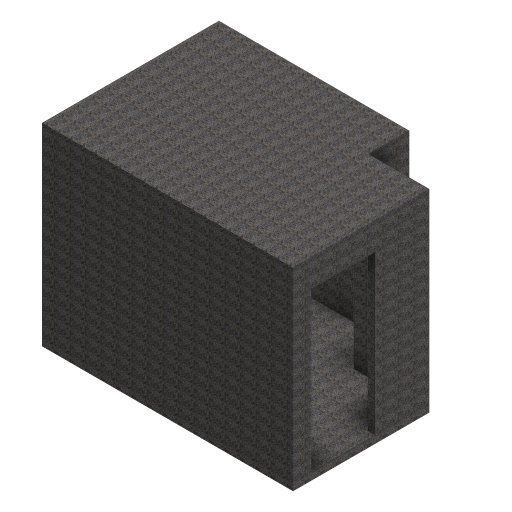
# Autodesk Inventor part: room
Saved by Autodesk Inventor 2023 (Build 270158000, 158)
## iProperties
Created: 2022-09-09
Part Number: room
Material: 混凝土
Document SubType Name: Modeling
Designer: byfbi
Density: 2.40731 g/cm^3
Appearance: 外露骨料 - 粗糙
Author: byfbi
Autodesk Inventor part; units mm, degrees
sketch "草图1" plane through (0, 0, 0) normal (0, 1, 0) x (-1, 0, 0)
  line L0 (0, 0) -> (0, 2400)
  line L1 (0, 2400) -> (-3500, 2400)
  line L2 (-3500, 2400) -> (-3500, 600)
  line L3 (-3500, 600) -> (-2600, 600)
  line L4 (-2600, 600) -> (-2600, 0)
  line L5 (-2600, 0) -> (0, 0)
  line L6 (110, 2510) -> (110, -110)
  line L7 (110, -110) -> (-2710, -110)
  line L8 (-2710, -110) -> (-2710, 490)
  line L9 (-2710, 490) -> (-3610, 490)
  line L10 (-3610, 490) -> (-3610, 2510)
  line L11 (-3610, 2510) -> (110, 2510)
  dimension "d0" = 2400
  dimension "d1" = 3500
  dimension "d2" = 1800
  dimension "d3" = 900
  dimension "d4" = 600
  dimension "d5" = 110
  constraints: 24 end point, 6 perpendicular, 2 vertical, 5 other
  measures "d0" distance of L0.start L0.end
  measures "d1" distance of L0.end L1.end
  measures "d2" distance of L1.end L2.end
  measures "d3" distance of L2.end L3.end
  measures "d4" distance of L3.end L4.end
  measures "d5" distance between parallel lines of L0 L6
extrude "拉伸1" add sketch "草图1" along normal blind 2650
sketch "草图2" plane through (0, 0, 0) normal (0, -1, 0) x (1, 0, 0)
  line L0 (3610, 2510) -> (3610, 490) projected
  line L1 (-110, 2510) -> (3610, 2510) projected
  line L2 (-110, -110) -> (-110, 2510) projected
  line L3 (2710, -110) -> (-110, -110) projected
  line L4 (2710, 490) -> (2710, -110) projected
  line L5 (3610, 490) -> (2710, 490) projected
  point P0 (0, 0)
extrude "拉伸2" add sketch "草图2" along normal blind 110
sketch "草图3" plane through (0, 2650, 0) normal (0, 1, 0) x (1, 0, 0)
  line L0 (-110, 110) -> (-110, -2510) projected
  line L1 (-110, -2510) -> (3610, -2510) projected
  line L2 (3610, -2510) -> (3610, -490) projected
  line L3 (3610, -490) -> (2710, -490) projected
  line L4 (2710, -490) -> (2710, 110) projected
  line L5 (2710, 110) -> (-110, 110) projected
  point P0 (0, 0)
extrude "拉伸3" add sketch "草图3" along normal blind 110
sketch "草图4" plane through (3610, -110, 2510) normal (1, 0, 0) x (0, 0, -1)
  line L0 (270, 2460) -> (1220, 2460)
  line L1 (1220, 2460) -> (1220, 110)
  line L2 (1220, 110) -> (270, 110)
  line L3 (270, 110) -> (270, 2460)
  line L4 (2020, 0) -> (2020, 2870) projected
  line L5 (0, 2870) -> (2020, 2870) projected
  point P0 (2510, 110)
  dimension "d12" = 950
  dimension "d13" = 2350
  dimension "d14" = 800
  dimension "d15" = 410
  constraints: 8 end point, 2 parallel, 1 horizontal, 1 perpendicular
  measures "d12" distance of L1.end L2.end
  measures "d13" distance of L0.end L1.end
  measures "d14" distance between parallel lines of L4 L1
  measures "d15" distance between parallel lines of L0 L5
extrude "拉伸4" cut sketch "草图4" against normal blind 110
sketch "草图5" plane through (0, 2760, 0) normal (0, 1, 0) x (1, 0, 0)
  line L0 (-110, -2510) -> (3610, -2510) projected
  line L1 (3610, -2510) -> (3610, -490) projected
  line L2 (3610, -490) -> (2710, -490) projected
  line L3 (2710, -490) -> (2710, 110) projected
  line L4 (2710, 110) -> (-110, 110) projected
  line L5 (-110, 110) -> (-110, -2510) projected
  point P0 (0, 0)
extrude "拉伸5" [suppressed]
ref_plane "工作平面1" through (2600, -110, 490) normal (1, 0, 0) x (0, 0, -1)
ref_plane "工作平面2" through (0, -110, -110) normal (-1, 0, 0) x (0, 0, 1)
ref_plane "工作平面3" through (2710, -110, 0) normal (0, 0, -1) x (-1, 0, 0)
ref_plane "工作平面4" through (0, 0, 0) normal (0, -1, 0) x (1, 0, 0)
ref_plane "工作平面5" through (-110, -110, 2400) normal (0, 0, 1) x (1, 0, 0)
ref_plane "工作平面6" through (1810, -110, 2510) normal (1, 0, 0) x (0, 0, -1)
ref_plane "工作平面7" through (0, 1500, 0) normal (0, -1, 0) x (1, 0, 0)
ref_plane "工作平面8" through (-110, -110, 1100) normal (0, 0, 1) x (1, 0, 0)
ref_plane "工作平面9" through (0, 2650, 0) normal (0, 1, 0) x (1, 0, 0)
ref_plane "工作平面10" through (3500, -110, 2510) normal (1, 0, 0) x (0, 0, -1)
sketch "草图6" plane through (3610, -110, 2510) normal (1, 0, 0) x (0, 0, -1)
  point P0 (2510, 110)
ref_plane "工作平面11" through (3610, -110, 2510) normal (1, 0, 0) x (0, 0, -1)
